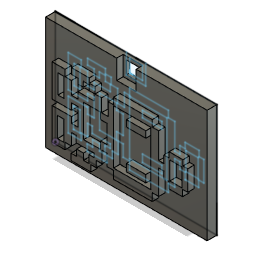
Keychain (Autodesk Fusion 360 design; units mm, degrees)
Autodesk Fusion 360 part; units mm, degrees
sketch "Sketch1" plane through (0, 0, 0) normal (0, 0, 1) x (1, 0, 0)
  line L0 (0, 0) -> (100, 0)
  line L1 (100, 0) -> (100, 70)
  line L2 (100, 70) -> (0, 70)
  line L3 (0, 70) -> (0, 0)
  line L4 (8, 52) -> (16, 52)
  line L5 (16, 52) -> (16, 48)
  line L6 (16, 48) -> (20, 48)
  line L7 (20, 48) -> (20, 40)
  line L8 (20, 40) -> (24, 40)
  line L9 (24, 40) -> (24, 44)
  line L10 (24, 44) -> (34, 44)
  line L11 (34, 44) -> (34, 48)
  line L12 (34, 48) -> (31.0135, 48)
  line L13 (31.0135, 48) -> (31.0135, 51.2095)
  line L14 (31.0135, 51.2095) -> (27.2594, 51.2095)
  line L15 (27.2594, 51.2095) -> (27.2594, 48)
  line L16 (27.2594, 48) -> (24, 48)
  line L17 (24, 48) -> (24, 51.2095)
  line L18 (24, 51.2095) -> (20, 51.2095)
  line L19 (20, 51.2095) -> (20, 54.8793)
  line L20 (20, 54.8793) -> (31.0135, 54.8793)
  line L21 (31.0135, 54.8793) -> (31.0135, 52)
  line L22 (31.0135, 52) -> (34.5568, 52)
  line L23 (34.5568, 52) -> (34.5568, 48)
  line L24 (34.5568, 48) -> (38.6062, 48)
  line L25 (38.6062, 48) -> (38.6062, 40)
  line L26 (38.6062, 40) -> (42.74, 40)
  line L27 (42.74, 40) -> (42.74, 48)
  line L28 (42.74, 48) -> (46, 48)
  line L29 (46, 48) -> (46, 52)
  line L30 (70, 52) -> (70, 48)
  line L31 (70, 48) -> (74, 48)
  line L32 (74, 48) -> (74, 32)
  line L33 (74, 32) -> (77.1603, 32)
  line L34 (77.1603, 32) -> (77.1603, 36.6146)
  line L35 (77.1603, 36.6146) -> (80.4082, 36.6146)
  line L36 (80.4082, 36.6146) -> (80.4082, 40)
  line L37 (80.4082, 40) -> (89.0133, 40)
  line L38 (89.0133, 40) -> (89.0133, 36.6146)
  line L39 (89.0133, 36.6146) -> (92, 36.6146)
  line L40 (92, 36.6146) -> (92, 24)
  line L41 (92, 24) -> (88.7602, 24)
  line L42 (88.7602, 24) -> (88.7602, 20)
  line L43 (88.7602, 20) -> (80.6613, 20)
  line L44 (80.6613, 20) -> (80.4082, 20)
  line L45 (80.4082, 20) -> (80.4082, 24)
  line L46 (80.4082, 24) -> (77.1603, 24)
  line L47 (77.1603, 24) -> (77.1603, 28)
  line L48 (77.1603, 28) -> (74, 28)
  line L49 (74, 28) -> (74, 12.7847)
  line L50 (74, 12.7847) -> (70, 12.7847)
  line L51 (70, 12.7847) -> (70, 8)
  line L52 (70, 8) -> (46, 8)
  line L53 (46, 8) -> (46, 12.7847)
  line L54 (46, 12.7847) -> (42, 12.7847)
  line L55 (42, 12.7847) -> (42, 20)
  line L56 (42, 20) -> (38.8928, 20)
  line L57 (38.8928, 20) -> (38.8928, 12.7847)
  line L58 (38.8928, 12.7847) -> (35.3422, 12.7847)
  line L59 (35.3422, 12.7847) -> (35.3422, 8.8329)
  line L60 (35.3422, 8.8329) -> (32, 8.8329)
  line L61 (32, 8.8329) -> (32, 4.8932)
  line L62 (32, 4.8932) -> (19.7075, 4.8932)
  line L63 (19.7075, 4.8932) -> (19.7075, 8.8329)
  line L64 (19.7075, 8.8329) -> (23.1089, 8.8329)
  line L65 (23.1089, 8.8329) -> (23.1089, 12.7847)
  line L66 (23.1089, 12.7847) -> (27.4055, 12.7847)
  line L67 (27.4055, 12.7847) -> (27.4055, 8.8329)
  line L68 (27.4055, 8.8329) -> (30.7472, 8.8329)
  line L69 (30.7472, 8.8329) -> (30.7472, 12.7847)
  line L70 (30.7472, 12.7847) -> (30.7472, 13.6069)
  line L71 (30.7472, 13.6069) -> (34, 13.6069)
  line L72 (34, 13.6069) -> (34, 16)
  line L73 (34, 16) -> (22.9001, 16)
  line L74 (22.9001, 16) -> (22.9001, 20)
  line L75 (22.9001, 20) -> (20, 20)
  line L76 (20, 20) -> (20, 13.1891)
  line L77 (20, 13.1891) -> (20, 12.8013)
  line L78 (20, 12.8013) -> (16, 12.8013)
  line L79 (16, 12.8013) -> (16, 8.8329)
  line L80 (16, 8.8329) -> (8, 8.8329)
  line L81 (8, 8.8329) -> (8, 28.5851)
  line L82 (8, 28.5851) -> (19.3793, 28.5851)
  line L83 (19.3793, 28.5851) -> (20, 28.5851)
  line L84 (20, 28.5851) -> (20, 24.9151)
  line L85 (20, 24.9151) -> (22.8106, 24.9151)
  line L86 (22.8106, 24.9151) -> (24, 24.9151)
  line L87 (24, 24.9151) -> (24, 36)
  line L88 (24, 36) -> (20, 36)
  line L89 (20, 36) -> (20, 32)
  line L90 (20, 32) -> (8, 32)
  line L91 (8, 32) -> (8, 52)
  line L92 (11.6437, 47.8919) -> (15.3019, 47.8919)
  line L93 (15.3019, 47.8919) -> (15.3019, 36)
  line L94 (15.3019, 36) -> (11.6437, 36)
  line L95 (11.6437, 36) -> (11.6437, 47.8919)
  line L96 (11.495, 24.9151) -> (15.3019, 24.9151)
  line L97 (15.3019, 24.9151) -> (15.3019, 12.4403)
  line L98 (15.3019, 12.4403) -> (11.6437, 12.4403)
  line L99 (11.6437, 12.4403) -> (11.2403, 12.4403)
  line L100 (11.2403, 12.4403) -> (11.2403, 24.9151)
  line L101 (11.2403, 24.9151) -> (11.495, 24.9151)
  line L102 (27.4611, 40) -> (27.4611, 20)
  line L103 (27.4611, 20) -> (38, 20)
  line L104 (38, 20) -> (38, 24.5326)
  line L105 (38, 24.5326) -> (42, 24.5326)
  line L106 (42, 24.5326) -> (42, 36)
  line L107 (42, 36) -> (38, 36)
  line L108 (38, 36) -> (38, 40)
  line L109 (38, 40) -> (27.4611, 40)
  line L110 (46.6458, 47.4856) -> (69.1094, 47.4856)
  line L111 (69.1094, 47.4856) -> (69.1094, 14)
  line L112 (69.1094, 14) -> (46, 14)
  line L113 (46, 14) -> (46, 47.4856)
  line L114 (46, 47.4856) -> (46.6458, 47.4856)
  line L115 (54, 44) -> (66, 44)
  line L116 (66, 44) -> (66, 40)
  line L117 (66, 40) -> (54, 40)
  line L118 (54, 40) -> (54, 44)
  line L119 (54, 20.5141) -> (66, 20.5141)
  line L120 (66, 20.5141) -> (66, 16)
  line L121 (66, 16) -> (54, 16)
  line L122 (54, 20.5141) -> (54, 16)
  line L123 (81.0563, 35.7923) -> (88.4585, 35.7923)
  line L124 (88.4585, 35.7923) -> (88.4585, 24.5409)
  line L125 (88.4585, 24.5409) -> (80.8786, 24.5409)
  line L126 (80.8786, 24.5409) -> (80.8786, 35.7923)
  line L127 (80.8786, 35.7923) -> (81.0563, 35.7923)
  line L128 (0, 70) -> (12, 70)
  line L129 (50, 70) -> (56, 70)
  line L130 (56, 70) -> (56, 58)
  line L131 (56, 58) -> (44, 58)
  line L132 (44, 58) -> (44, 70)
  line L133 (46, 68) -> (54, 68)
  line L134 (54, 68) -> (54, 60)
  line L135 (54, 60) -> (46, 60)
  line L136 (46, 60) -> (46, 68)
  line L137 (46, 52) -> (70, 52)
  dimension "d1" = 100
  dimension "d2" = 70
  constraint horizontal L0
  constraint vertical L1
  constraint horizontal L2
  constraint vertical L3
  constraint coincident L0.start L3.end
  constraint horizontal L4
  constraint perpendicular L4 L5
  constraint perpendicular L5 L6
  constraint perpendicular L6 L7
  constraint perpendicular L7 L8
  constraint perpendicular L8 L9
  constraint perpendicular L9 L10
  constraint perpendicular L10 L11
  constraint perpendicular L11 L12
  constraint perpendicular L12 L13
  constraint perpendicular L13 L14
  constraint perpendicular L14 L15
  constraint perpendicular L13 L16
  constraint perpendicular L14 L17
  constraint perpendicular L17 L18
  constraint perpendicular L18 L19
  constraint perpendicular L13 L20
  constraint perpendicular L14 L21
  constraint perpendicular L11 L22
  constraint perpendicular L12 L23
  constraint perpendicular L23 L24
  constraint perpendicular L24 L25
  constraint perpendicular L25 L26
  constraint perpendicular L26 L27
  constraint perpendicular L25 L28
  constraint perpendicular L28 L29
  constraint perpendicular L28 L30
  constraint perpendicular L30 L31
  constraint perpendicular L31 L32
  constraint perpendicular L32 L33
  constraint perpendicular L31 L34
  constraint perpendicular L34 L35
  constraint perpendicular L35 L36
  constraint perpendicular L34 L37
  constraint perpendicular L37 L38
  constraint perpendicular L38 L39
  constraint perpendicular L39 L40
  constraint perpendicular L40 L41
  constraint perpendicular L39 L42
  constraint perpendicular L42 L43
  constraint perpendicular L36 L44
  constraint perpendicular L43 L45
  constraint perpendicular L34 L46
  constraint perpendicular L33 L47
  constraint perpendicular L47 L48
  constraint perpendicular L48 L49
  constraint perpendicular L49 L50
  constraint perpendicular L50 L51
  constraint perpendicular L51 L52
  constraint perpendicular L52 L53
  constraint perpendicular L53 L54
  constraint perpendicular L54 L55
  constraint perpendicular L55 L56
  constraint perpendicular L56 L57
  constraint perpendicular L57 L58
  constraint perpendicular L58 L59
  constraint perpendicular L57 L60
  constraint perpendicular L60 L61
  constraint perpendicular L61 L62
  constraint perpendicular L62 L63
  constraint perpendicular L63 L64
  constraint perpendicular L58 L65
  constraint perpendicular L65 L66
  constraint perpendicular L60 L67
  constraint perpendicular L67 L68
  constraint perpendicular L60 L69
  constraint perpendicular L60 L70
  constraint perpendicular L70 L71
  constraint perpendicular L71 L72
  constraint perpendicular L72 L73
  constraint perpendicular L71 L74
  constraint perpendicular L74 L75
  constraint perpendicular L75 L76
  constraint perpendicular L75 L77
  constraint perpendicular L65 L78
  constraint perpendicular L64 L79
  constraint perpendicular L79 L80
  constraint perpendicular L80 L81
  constraint perpendicular L81 L82
  constraint perpendicular L81 L83
  constraint perpendicular L83 L84
  constraint perpendicular L84 L85
  constraint perpendicular L9 L86
  constraint perpendicular L86 L87
  constraint perpendicular L87 L88
  constraint perpendicular L86 L89
  constraint perpendicular L89 L90
  constraint perpendicular L4 L91
  constraint horizontal L92
  constraint perpendicular L92 L93
  constraint perpendicular L93 L94
  constraint perpendicular L92 L95
  constraint perpendicular L93 L96
  constraint perpendicular L78 L97
  constraint perpendicular L97 L98
  constraint perpendicular L97 L99
  constraint perpendicular L96 L100
  constraint parallel L96 L101
  constraint perpendicular L75 L102
  constraint perpendicular L102 L103
  constraint perpendicular L103 L104
  constraint perpendicular L102 L105
  constraint perpendicular L105 L106
  constraint perpendicular L106 L107
  constraint perpendicular L105 L108
  constraint perpendicular L106 L109
  constraint perpendicular L106 L110
  constraint perpendicular L31 L111
  constraint perpendicular L106 L112
  constraint perpendicular L110 L113
  constraint perpendicular L113 L114
  constraint perpendicular L113 L115
  constraint perpendicular L115 L116
  constraint perpendicular L116 L117
  constraint perpendicular L115 L118
  constraint perpendicular L118 L119
  constraint perpendicular L115 L120
  constraint perpendicular L120 L121
  constraint perpendicular L121 L122
  constraint perpendicular L49 L123
  constraint perpendicular L46 L124
  constraint perpendicular L124 L125
  constraint perpendicular L46 L126
  constraint perpendicular L126 L127
  constraint coincident L2 L128.end
  constraint midpoint L2 L129.start
  constraint coincident L2 L129.end
  constraint perpendicular L2 L130
  constraint perpendicular L130 L131
  constraint coincident L2 L132.end
  constraint perpendicular L2 L132
  constraint perpendicular L133 L134
  constraint perpendicular L134 L135
  constraint perpendicular L133 L136
  constraint perpendicular L30 L137
  measures "d1" distance of L0.start L0.end
  measures "d2" distance of L0.start L2.end
extrude "Extrude1" add sketch "Sketch1" along normal blind 2 makes body 1 at (13.948, 16.5986, 0) makes body 2 at (74.6667, 63.3333, 0) makes body 3 at (62, 27.0094, 0) makes body 4 at (12.8631, 43.928, 0) makes body 5 at (30.9741, 28.1775, 0) makes body 6 at (85.9319, 28.2914, 0)
extrude "Extrude2" add sketch "Sketch1" along normal blind 10 contours L4 L5 L6 L7 L8 L9 L10 L11 L12 L13 L14 L15 L16 L17 L18 L19 L20 L21 L22 L23 L24 L25 L26 L27 L28 L29 L30 L31 L32 L33 L34 L35 L36 L37 L38 L39 L40 L41 L42 L43 L44 L45 L46 L47 L48 L49 L50 L51 L52 L53 L54 L55 L56 L57 L58 L59 L60 L61 L62 L63 L64 L65 L66 L67 L68 L69 L70 L71 L72 L73 L74 L75 L76 L77 L78 L79 L80 L81 L82 L83 L84 L85 L86 L87 L88 L89 L90 L91 L137 | L115 L116 L117 L118 | L119 L120 L121 L122 bodies 1 2 3 4 5 6
extrude "Extrude3" add 6 faces at (74.6667, 63.3333, 2) (62, 27.0094, 2) (85.9319, 28.2914, 2) (30.9741, 28.1775, 2) (12.8631, 43.928, 2) (13.948, 16.5986, 2) along direction (0, 0, 1) blind 4 on bodies 1 bodies 1
extrude "Extrude4" cut sketch "Sketch1" along normal blind 11 contours L2 L129 L130 L131 L132 bodies 1
extrude "Extrude5" add sketch "Sketch1" along normal blind 2 contours L2 L129 L130 L131 L132 bodies 1
named bodies: "Keychain 2 - Robot"
